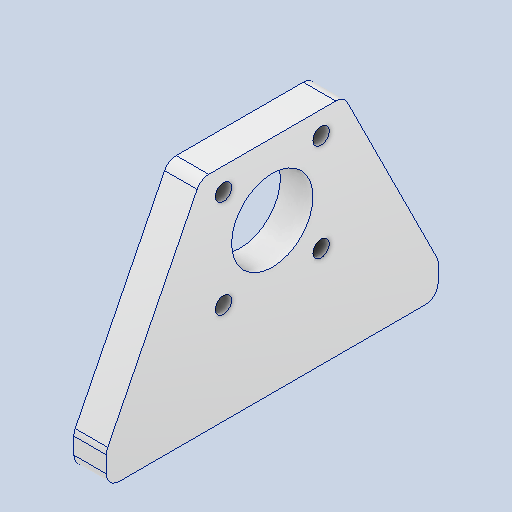
# Autodesk Inventor part: belt_liner_v2_Plate_21
Saved by Autodesk Inventor 2025.2 (Build 292293000, 293)
## iProperties
Created: 2025-01-28
Part Number: belt_liner_v2_Plate_21
Material: アルミニウム 6061
Document SubType Name: Modeling
Designer: haruy
Density: 2.7 g/cm^3
Appearance: アルミニウム - フラット
Author: haruy
Autodesk Inventor part; units mm, degrees
ref_plane "YZ Plane" through (0, 0, 0) normal (1, 0, 0) x (0, 1, 0)
ref_plane "XZ Plane" through (0, 0, 0) normal (0, 1, 0) x (-1, 0, 0)
ref_plane "XY Plane" through (0, 0, 0) normal (0, 0, 1) x (1, 0, 0)
sketch "スケッチ1" plane through (0, 0, 0) normal (1, 0, 0) x (0, 1, 0)
  line L0 (0, 0) -> (15, 0)
  line L1 (15, 0) -> (15, -15)
  line L2 (15, -15) -> (0, -15)
  line L3 (0, -15) -> (0, 0)
  line L4 (0, 18) -> (-5, 18)
  line L5 (-5, 18) -> (-5, -33)
  line L6 (-5, -33) -> (0, -33)
  line L7 (0, -33) -> (0, 18)
  line L8 (12, 3.5) -> (34, 3.5)
  line L9 (34, 3.5) -> (34, -18.5)
  line L10 (34, -18.5) -> (12, -18.5)
  line L11 (12, -18.5) -> (12, 3.5)
  circle A0 centre (15.5, 0) radius 1.25
  line L12 (23, 3.5) -> (23, -18.5)
  line L13 (34, -7.5) -> (12, -7.5)
  circle A1 centre (15.5, -15) radius 1.25
  circle A2 centre (30.5, 0) radius 1.25
  circle A3 centre (30.5, -15) radius 1.25
  circle A4 centre (23, -7.5) radius 6.25
  line L14 (0, 18) -> (34, 3.5)
  line L15 (34, -18.5) -> (0, -33)
  line L16 (0, 18) -> (5, 18)
  line L17 (5, 18) -> (34, 3.5)
  line L18 (0, -33) -> (5, -33)
  line L19 (5, -33) -> (34, -18.5)
  dimension "d0" = 15
  dimension "d1" = 15
  dimension "d2" = 5
  dimension "d3" = 51
  dimension "d4" = 18
  dimension "d5" = 0
  dimension "d6" = 22
  dimension "d7" = 22
  dimension "d8" = 3.5
  dimension "d9" = 3
  dimension "d10" = 2.5
  dimension "d11" = 3.5
  dimension "d12" = 3.5
  dimension "d13" = 12.5
  dimension "d18" = 5
  constraints: 40 end point, 6 parallel, 5 centre point, 5 midpoint, 4 horizontal, 4 symmetric about line, 3 perpendicular, 3 other
  measures "d0" distance of L1.end L2.end
  measures "d1" distance of L0.end L1.end
  measures "d2" distance of L6.end L5.end
  measures "d3" distance between parallel lines of L6 L4
  measures "d4" distance between parallel lines of L0 L4
  measures "d5" distance between parallel lines of L7 L3
  measures "d6" distance of L9.end L10.end
  measures "d7" distance of L8.end L9.end
  measures "d8" distance between parallel lines of L0 L8
  measures "d9" distance between parallel lines of L1 L11
  measures "d10" diameter of A0
  measures "d11" distance from line of A0.centre L11
  measures "d12" distance from line of A0.centre L8
  measures "d13" diameter of A4
  measures "d18" distance of L4.start L16.end
extrude "押し出し1" add sketch "スケッチ1" against normal blind 5 contours L7 L14 L8 L11 L0 | L0 L11 L2 L3 | L11 L8 L12 A4 L13 L1 A0 L0 | L0 A0 L1 L13 L11 | L2 L11 L10 L15 L7 | L16 L17 L14 | L13 L1 A1 L2 L11 | L2 A1 L1 L13 A4 L12 L10 L11 | L15 L19 L18 | L9 L13 A4 L12 L8 | L10 L12 A4 L13 L9
fillet "フィレット2" radius 2 6 edges at (-2.5, 0, -33) (-2.5, 5, -33) (-2.5, 34, -18.5) (-2.5, 34, 3.5) (-2.5, 0, 18) (-2.5, 5, 18)
sketch "スケッチ3" plane through (0, 0, -31) normal (0, -1, 0) x (1, 0, 0)
  line L0 (0, 29.75) -> (0, 17.25) projected
  line L1 (0, 23.5) -> (-5, 23.5)
  line L2 (-5, 17.25) -> (-5, 29.75) projected
  line L3 (0, 47) -> (0, 0) projected
  line L4 (0, 33.5) -> (-5, 33.5)
  line L5 (0, 13.5) -> (-5, 13.5)
  point P0 (0, 31)
  point P1 (-2.5, 33.5)
  point P2 (-2.5, 23.5)
  point P3 (-2.5, 13.5)
  dimension "d20" = 10
  dimension "d21" = 2.5
  dimension "d22" = 2.5
  constraints: 6 end point, 5 midpoint, 2 symmetric about line, 1 horizontal, 1 point on line
  measures "d20" distance between parallel lines of L4 L1
  measures "d21" distance from line of point (-2.5, 13.5) L2
  measures "d22" distance from line of point (-2.5, 33.5) L2
hole "穴1" at (-2.5, 0, 2.5) at (-2.5, 0, -7.5) at (-2.5, 0, -17.5) direction (0, 1, 0) diameter 2.5 depth 5 tip angle 118
